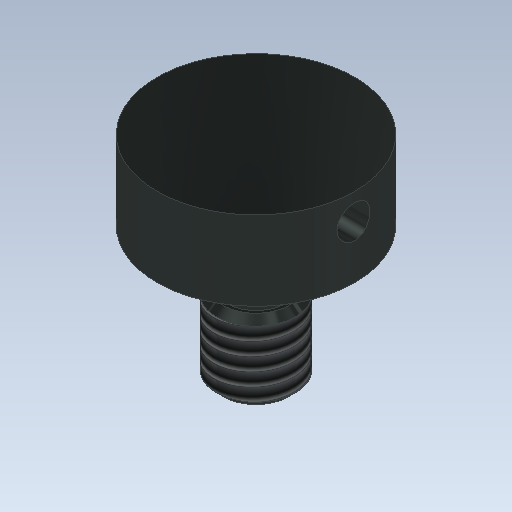
# Autodesk Inventor part: Thumb Screw
Saved by Autodesk Inventor 2020 (Build 240168000, 168)
## iProperties
Created: 2012-10-13
Part Number: Thumb Screw
Material: Steel, Mild
Document SubType Name: Modeling
Designer: Lance
Mass: 10.5349 g
Surface Area: 9.46241 cm^2
Volume: 1.34031 cm^3
Density: 7.86 g/cm^3
Appearance: Gunmetal - Polished
Author: Lance
Autodesk Inventor part; units mm, degrees
ref_plane "YZ Plane" through (0, 0, 0) normal (1, 0, 0) x (0, 1, 0)
ref_plane "XZ Plane" through (0, 0, 0) normal (0, 1, 0) x (-1, 0, 0)
ref_plane "XY Plane" through (0, 0, 0) normal (0, 0, 1) x (1, 0, 0)
sketch "Sketch3" plane through (0, 0, 0) normal (0, 0, 1) x (1, 0, 0)
  line L0 (0, 3) -> (7.5, 3)
  line L1 (7.5, 3) -> (7.5, -3)
  line L2 (7.5, -3) -> (4.5, -3)
  line L3 (4.5, -3) -> (4.5, -5)
  line L4 (4.5, -5) -> (3, -5)
  line L5 (0, -16.2) -> (0, 6.2) projected
  line L6 (3, -5) -> (3, -13)
  line L7 (3, -13) -> (0, -13)
  point P0 (0, 0)
  point P1 (7.5, 0)
  dimension "d6" = 6
  dimension "d7" = 15
  dimension "d8" = 9
  dimension "d9" = 2
  dimension "d11" = 6
  dimension "d12" = 8
  constraints: 14 end point, 4 parallel, 2 perpendicular, 2 point on line, 1 horizontal, 1 horizontal alignment, 1 midpoint
  measures "d6" distance between parallel lines of L2 L0
  measures "d7" diameter of L1 L5
  measures "d8" diameter of L3 L5
  measures "d9" distance between parallel lines of L2 L4
  measures "d11" diameter of L6 L5
  measures "d12" distance between parallel lines of L4 L7
revolve "Revolution1" add sketch "Sketch3" angle 360 about axis through (0, -10, 0) along (0, 1, 0)
sketch "Sketch4" plane through (0, 0, 0) normal (1, 0, 0) x (0, 1, 0)
  circle A0 centre (1, 0) radius 1.25
  line L0 (3, 7.5) -> (3, -7.5) projected
  point P0 (0, 0)
  dimension "d13" = 2.5
  dimension "d14" = 2
  constraints: 1 centre point, 1 horizontal alignment
  measures "d13" diameter of A0
  measures "d14" distance from line of A0.centre L0
extrude "Extrusion3" cut sketch "Sketch4" along normal through all both and the other way through all
sketch "Sketch5" plane through (0, 0, 0) normal (1, 0, 0) x (0, 1, 0)
  line L0 (-7, 2.25) -> (-5, 2.25)
  line L1 (-5, 2.25) -> (-5, 3)
  line L2 (-5, 3) -> (-7, 3)
  line L3 (-7, 3) -> (-7, 2.25)
  line L4 (-5, 3) -> (-13, 3) projected
  line L5 (-5, 4.5) -> (-5, -4.5) projected
  line L6 (-16.2, 0) -> (6.2, 0) projected
  point P0 (0, 0)
  dimension "d17" = 2
  dimension "d18" = 4.5
  constraints: 8 end point, 2 collinear, 2 parallel, 1 horizontal, 1 perpendicular
  measures "d17" distance between parallel lines of L1 L3
  measures "d18" diameter of L0 L6
revolve "Revolution2" cut sketch "Sketch5" angle 360 about axis through (0, -10, 0) along (0, 1, 0)
thread "Thread1" size "M6x1" class "6g" standard "ANSI Metric M Profile" full length
chamfer "Chamfer1" distance 0.5 angle 45 2 edges at (-3, -13, 0) (-3, -7, 0)
body "Solid2"
